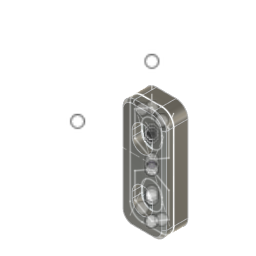
[a]_z_chain_retainer_bracket_x2 (Autodesk Fusion 360 design; units mm, degrees)
Autodesk Fusion 360 part; units mm, degrees
note: some values were not read from the file. Set by a fixed rule: which sketch regions a step uses.
sketch "Sketch1" plane through (0, 0, 0) normal (0, 1, 0) x (1, 0, 0)
  line L0 (-1.65, 9.2209) -> (1.65, 9.2209)
  line L1 (3.65, 7.2209) -> (3.65, -7.2209)
  line L2 (1.65, -9.2209) -> (-1.65, -9.2209)
  line L3 (-3.65, -7.2209) -> (-3.65, 7.2209)
  line L4 (-3.65, 9.2209) -> (3.65, -9.2209) construction
  line L5 (3.65, 9.2209) -> (-3.65, -9.2209) construction
  line L6 (0, 0) -> (0, -15) construction
  line L7 (0, 0) -> (-12.5, 0) construction
  line L8 (1.7, -5) -> (1.7, -4)
  arc A0 (1.7, -4) -> (-1.7, -4) centre (0, -4) ccw
  line L9 (-1.7, -4) -> (-1.7, -5)
  arc A1 (-1.7, -5) -> (1.7, -5) centre (0, -5) ccw
  line L10 (0, -5) -> (0, -4) construction
  line L11 (0, -8.2909) -> (2.85, -6.6454)
  line L12 (2.85, -6.6454) -> (2.85, -2.3546)
  line L13 (2.85, -2.3546) -> (0, -0.7091)
  line L14 (0, -8.2909) -> (-2.85, -6.6454)
  line L15 (-2.85, -6.6454) -> (-2.85, -2.3546)
  line L16 (-2.85, -2.3546) -> (0, -0.7091)
  line L17 (0, -5) -> (-2.85, -6.6454) construction
  line L18 (0, -4) -> (-2.85, -2.3546) construction
  line L19 (0, 8.2909) -> (-2.85, 6.6454)
  line L20 (-2.85, 6.6454) -> (-2.85, 2.3546)
  line L21 (-2.85, 2.3546) -> (0, 0.7091)
  line L22 (2.85, 2.3546) -> (0, 0.7091)
  line L23 (2.85, 6.6454) -> (2.85, 2.3546)
  line L24 (0, 8.2909) -> (2.85, 6.6454)
  arc A2 (1.7, 5) -> (-1.7, 5) centre (0, 5) ccw
  line L25 (-1.7, 4) -> (-1.7, 5)
  arc A3 (-1.7, 4) -> (1.7, 4) centre (0, 4) ccw
  line L26 (1.7, 5) -> (1.7, 4)
  arc A4 (-3.65, -7.2209) -> (-1.65, -9.2209) centre (-1.65, -7.2209) ccw
  arc A5 (-1.65, 9.2209) -> (-3.65, 7.2209) centre (-1.65, 7.2209) ccw
  arc A6 (3.65, 7.2209) -> (1.65, 9.2209) centre (1.65, 7.2209) ccw
  arc A7 (1.65, -9.2209) -> (3.65, -7.2209) centre (1.65, -7.2209) ccw
  point P0 (0, -4.5)
  point P1 (0, 4.5)
  dimension "d2" = 1.7
  dimension "d4" = 1
  dimension "d5" = 120
  dimension "d6" = 120
  dimension "d8" = 5.7
  dimension "d10" = 60
  dimension "d11" = 60
  dimension "d12" = 9
  dimension "d13" = 0.93
  dimension "d14" = 0.8
  dimension "d19" = 2
  constraint horizontal L0
  constraint perpendicular L0 L1
  constraint parallel L0 L2
  constraint parallel L1 L3
  constraint coincident L4 L6.start
  constraint coincident L5 L6.start
  constraint coincident L6.start L7.start
  constraint parallel L3 L6
  constraint perpendicular L6 L7
  constraint tangent L8 A0
  constraint tangent A0 L9
  constraint parallel L8 L9
  constraint tangent L9 A1
  constraint tangent L8 A1
  constraint coincident L6 A0.centre
  constraint parallel L6 L10
  constraint coincident L6 L11.start
  constraint parallel L6 L12
  constraint coincident L6 L13.end
  constraint symmetric L6 L11.start L14.start
  constraint symmetric L6 L11.end L14.end
  constraint symmetric L6 L12.end L15.end
  constraint symmetric L6 L13.end L16.end
  constraint midpoint L10 P0
  constraint coincident A1.centre L10.start
  constraint coincident A0.centre L10.end
  constraint symmetric L7 L8.start A2.start
  constraint symmetric L7 L8.end A3.end
  constraint symmetric L7 A0.end L25.start
  constraint symmetric L7 L9.end A2.end
  constraint symmetric L7 A0 A3
  constraint symmetric L7 A1 A2
  constraint symmetric L7 L11.start L19.start
  constraint symmetric L7 L11.end L23.start
  constraint symmetric L7 L12.end L22.start
  constraint symmetric L7 L13.end L21.end
  constraint symmetric L7 L14.end L19.end
  constraint symmetric L7 L15.end L20.end
  constraint symmetric L7 P0 P1
  constraint coincident L5.end L2
  constraint coincident L5.end L3
  constraint tangent L2 A4
  constraint tangent L3 A4
  constraint coincident L4.start L3
  constraint coincident L4.start L0
  constraint tangent L3 A5
  constraint tangent L0 A5
  constraint equal A4 A5
  constraint coincident L5.start L0
  constraint coincident L5.start L1
  constraint tangent L0 A6
  constraint tangent L1 A6
  constraint equal A4 A6
  constraint coincident L4.end L1
  constraint coincident L4.end L2
  constraint tangent L1 A7
  constraint tangent L2 A7
  constraint equal A4 A7
  measures "d2" radius of A1
  measures "d4" distance of A1.centre A0.centre
  measures "d5" angle of L11 L12
  measures "d6" angle of L12 L13
  measures "d8" distance of L12 L15
  measures "d10" angle of L14 L17
  measures "d11" angle of L16 L18
  measures "d12" distance of P0 P1
  measures "d13" distance of L2 L11.start
  measures "d14" distance of L1 L12
  measures "d19" radius of A4
extrude "Extrude1" add sketch "Sketch1" along normal blind 2.4 contours L0 L1 L2 L3 A4 A5 A6 A7
extrude "Extrude2" add sketch "Sketch1" against normal blind 1.6 contours L0 L1 L2 L3 A4 A5 A6 A7 | L11 L12 L13 L14 L15 L16 | L19 L20 L21 L22 L23 L24
chamfer "Chamfer1" distance 0.4 angle 45 8 edges at (-3.0642, -1.6, 8.6351) (-3.65, -1.6, 0) (-3.0642, -1.6, -8.6351) (0, -1.6, -9.2209) (3.0642, -1.6, -8.6351) (3.65, -1.6, 0) (3.0642, -1.6, 8.6351) (0, -1.6, 9.2209)
equation "hole_diameter = 3.4 mm"
equation "d2 = hole_diameter / 2"
equation "screw_travel = 1 mm"
equation "d4 = screw_travel"
